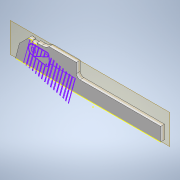
# Autodesk Inventor part: FINALcASEING
Saved by Autodesk Inventor 2022 (Build 260153000, 153)
## iProperties
Created: 2022-05-17
Part Number: FINALcASEING
Material: Generic
Document SubType Name: Sheet Metal
Designer: joshn
Density: 1 g/cm^3
Sheet Metal Rule: Default
Appearance: Default
Author: joshn
Autodesk Inventor part; units mm, degrees
ref_plane "YZ Plane" through (0, 0, 0) normal (1, 0, 0) x (0, 1, 0)
ref_plane "XZ Plane" through (0, 0, 0) normal (0, 1, 0) x (-1, 0, 0)
ref_plane "XY Plane" through (0, 0, 0) normal (0, 0, 1) x (1, 0, 0)
sketch "Sketch1" plane through (0, 0, 0) normal (0, 0, 1) x (1, 0, 0)
  line L0 (26.0925, 1.395) -> (-29.8488, 1.395)
  line L1 (26.0925, 6.611) -> (26.0925, 1.395)
  line L2 (-4.9967, 6.611) -> (26.0925, 6.611)
  arc A0 (-6.3815, 7.9958) -> (-4.9967, 6.611) centre (-4.9967, 7.9958) ccw
  line L3 (-6.3815, 11.7522) -> (-6.3815, 7.9958)
  arc A1 (2.6948, 11.4852) -> (3.6377, 11.1665) centre (3.6377, 12.7207) ccw
  line L4 (28.1816, 11.1665) -> (3.6377, 11.1665)
  arc A2 (28.1816, 11.1665) -> (28.7773, 11.4852) centre (28.1816, 11.8825) ccw
  line L5 (33.3358, 11.4852) -> (28.7773, 11.4852)
  line L6 (33.3358, 4.3481) -> (33.3358, 11.4852)
  line L7 (31.5081, -0.0048) -> (33.3358, 4.3481)
  line L8 (6.4399, -0.0048) -> (31.5081, -0.0048)
  arc A3 (6.4399, -0.0048) -> (0.2019, -8.5692) centre (6.4399, -6.5588) ccw
  arc A4 (-0.2259, -9.1565) -> (0.2019, -8.5692) centre (-0.2259, -8.7071) ccw
  line L9 (-8.1638, -9.1565) -> (-0.2259, -9.1565)
  line L10 (-9.2556, -8.793) -> (-8.1638, -9.1565)
  arc A5 (-9.2556, -8.793) -> (-11.9702, -10.6446) centre (-9.6874, -11.0757) ccw
  line L11 (-14.0648, -21.738) -> (-11.9702, -10.6446)
  arc A6 (-14.0648, -21.738) -> (-13.9231, -23.1489) centre (-11.5297, -22.1959) ccw
  line L12 (-12.9221, -25.6631) -> (-13.9231, -23.1489)
  line L13 (-29.6181, -25.6631) -> (-12.9221, -25.6631)
  line L14 (-30.9465, -25.0614) -> (-29.6181, -25.6631)
  line L15 (-31.1458, -21.5976) -> (-30.9465, -25.0614)
  arc A7 (-30.2453, -17.6448) -> (-31.1458, -21.5976) centre (-23.86, -21.1784) ccw
  arc A8 (-30.2453, -17.6448) -> (-27.8942, -12.0594) centre (-55.0684, -3.9079) ccw
  line L16 (-26.4293, -7.1761) -> (-27.8942, -12.0594)
  arc A9 (-26.4293, -7.1761) -> (-31.0096, -1.0202) centre (-31.0096, -5.8021) ccw
  line L17 (-36.2536, -1.0202) -> (-31.0096, -1.0202)
  arc A10 (-36.381, -0.6693) -> (-36.2536, -1.0202) centre (-36.2536, -0.8216) ccw
  arc A11 (-31.0437, 1.6032) -> (-36.381, -0.6693) centre (-29.9586, -8.349) ccw
  line L18 (-28.3022, 7.1894) -> (-29.8488, 1.395)
  arc A12 (-8.4832, -1.7741) -> (-7.3734, -1.1742) centre (-9.8084, 2.0038) ccw
  arc A13 (-8.4832, -1.7741) -> (-9.7826, -7.4755) centre (-7.34, -5.0334) ccw
  arc A14 (-9.7826, -7.4755) -> (-7.6044, -8.3792) centre (-7.6013, -5.2947) ccw
  line L19 (-7.6044, -8.3792) -> (-2.3274, -8.3792)
  arc A15 (-2.3274, -8.3792) -> (-1.0505, -7.1023) centre (-2.3274, -7.1023) ccw
  line L20 (-1.0505, -7.1023) -> (-1.0505, -4.8739)
  arc A16 (-1.0505, -4.8739) -> (-4.9041, -1.0202) centre (-4.9041, -4.8739) ccw
  line L21 (-4.9041, -1.0202) -> (-6.9193, -1.0202)
  arc A17 (-6.9193, -1.0202) -> (-7.3734, -1.1742) centre (-6.9193, -1.767) ccw
  arc A18 (-19.7638, 10.6339) -> (-16.9019, 11.7522) centre (-19.7638, 14.8551) ccw
  line L22 (-6.3815, 11.7522) -> (-16.9019, 11.7522)
  line L23 (-19.7638, 10.6339) -> (-21.6251, 10.6339)
  line L24 (-23.3493, 10.6339) -> (-24.8791, 10.6339)
  line L25 (-24.8791, 10.6339) -> (-28.3022, 7.1894)
  line L26 (-23.3493, 10.6339) -> (-23.7221, 10.0493)
  line L27 (-23.7221, 10.0493) -> (-21.2622, 10.0493)
  line L28 (-21.2622, 10.0493) -> (-21.6251, 10.6339)
  point P0 (0, 0)
extrude "Plate1" add sketch "Sketch1" along normal blind 1.5 contours L0 L18 L25 L24 L26 L27 L28 L23 A18 L22 L3 A0 L2 L1
sketch "Sketch2" plane through (0, 0, 1.5) normal (0, 0, 1) x (1, 0, 0)
  line L0 (-24.8791, 10.6339) -> (-23.3493, 10.6339) projected
  line L1 (-24.2815, 10.6339) -> (-26.8252, 1.395)
  line L2 (26.0925, 1.395) -> (-29.8488, 1.395) projected
  line L3 (-16.1938, 8.4071) -> (-18.7375, -0.8317)
  line L4 (-15.9942, 8.3522) -> (-18.5379, -0.8867)
  line L5 (-15.2196, 8.1389) -> (-17.7634, -1.1)
  line L6 (-14.9385, 8.0615) -> (-17.4822, -1.1774)
  line L7 (-13.9643, 7.7933) -> (-16.5081, -1.4456)
  line L8 (-13.7067, 7.7224) -> (-16.2504, -1.5165)
  line L9 (-12.8263, 7.48) -> (-15.37, -1.7589)
  line L10 (-12.5495, 7.4038) -> (-15.0932, -1.8351)
  line L11 (-11.612, 7.1457) -> (-14.1558, -2.0932)
  line L12 (-11.4028, 7.0881) -> (-13.9465, -2.1508)
  line L13 (-10.3931, 6.8101) -> (-12.9369, -2.4288)
  line L14 (-10.137, 6.7395) -> (-12.6808, -2.4993)
  line L15 (-9.1755, 6.4748) -> (-11.7192, -2.7641)
  line L16 (-8.9034, 6.3999) -> (-11.4471, -2.839)
  line L17 (-8.1272, 6.2147) -> (-10.7056, -3.1502)
  line L18 (-7.8808, 6.2147) -> (-10.4766, -3.2133)
  line L19 (-6.8145, 6.2147) -> (-9.4855, -3.4861)
  line L20 (-6.9417, 6.2147) -> (-9.6037, -3.4536)
  arc A0 (-22.976, 9.5181) -> (-23.3371, 5.5802) centre (-23.0061, 7.5354) ccw
  line L21 (-22.976, 9.5181) -> (-17.7655, 9.5181)
  arc A1 (-16.95, 8.7307) -> (-17.7655, 9.5181) centre (-17.7655, 8.7021) ccw
  line L22 (-16.95, 8.7307) -> (-16.8802, 6.7415)
  line L23 (-16.8802, 6.7415) -> (-17.3174, 5.1538)
  arc A2 (-18.0525, 4.6855) -> (-17.3174, 5.1538) centre (-17.944, 5.3263) ccw
  line L24 (-18.0525, 4.6855) -> (-23.3371, 5.5802)
  circle A3 centre (-23.0061, 7.5354) radius 0.8711
  arc A4 (-23.0061, 9.3529) -> (-22.235, 5.8895) centre (-23.0061, 7.5354) ccw
  line L25 (-23.0061, 9.3529) -> (-17.7655, 9.3529)
  arc A5 (-17.4894, 8.1128) -> (-17.7655, 9.3529) centre (-17.7655, 8.7021) ccw
  line L26 (-17.4894, 8.1128) -> (-22.235, 5.8895)
  line L27 (-6.8145, 6.2147) -> (-17.0253, 6.2147)
  line L28 (-23.3493, 10.6339) -> (-23.7221, 10.0493) projected
  line L29 (-23.7221, 10.0493) -> (-21.2622, 10.0493) projected
  line L30 (-22.2015, 5.818) -> (-17.4559, 8.0413)
  arc A6 (-17.4559, 8.0413) -> (-17.7655, 9.4318) centre (-17.7655, 8.7021) ccw
  line L31 (-17.7655, 9.4318) -> (-23.0061, 9.4318)
  arc A7 (-23.0061, 9.4318) -> (-22.2015, 5.818) centre (-23.0061, 7.5354) ccw
  line L32 (-22.9381, 6.6239) -> (-23.0741, 6.6239)
  line L33 (-23.0741, 6.6239) -> (-23.0741, 8.4468)
  line L34 (-23.0741, 8.4468) -> (-22.9381, 8.4468)
  line L35 (-22.9381, 8.4468) -> (-22.9381, 6.6239)
  line L36 (-22.9381, 6.6239) -> (-23.0741, 8.4468) construction
  line L37 (-23.0741, 6.6239) -> (-22.9381, 8.4468) construction
  line L38 (-23.2868, 10.36) -> (-23.5907, 9.2563)
  line L39 (-23.0483, 10.2944) -> (-23.858, 7.3534)
  line L40 (-24.3892, 6.3561) -> (-24.4143, 6.265)
  line L41 (-24.4413, 6.1669) -> (-25.8305, 1.1212)
  line L42 (-24.188, 6.1546) -> (-24.2111, 6.0709)
  line L43 (-24.2361, 5.9799) -> (-25.592, 1.0555)
  line L44 (-22.1805, 10.0555) -> (-23.386, 5.6773)
  line L45 (-23.409, 5.5937) -> (-24.7242, 0.8166)
  line L46 (-21.9016, 9.9786) -> (-23.0959, 5.641)
  line L47 (-23.1226, 5.5439) -> (-24.4453, 0.7398)
  line L48 (-20.9546, 9.7179) -> (-22.0026, 5.9112)
  line L49 (-22.1492, 5.379) -> (-23.4983, 0.479)
  line L50 (-20.7608, 9.6646) -> (-21.7633, 6.0233)
  line L51 (-21.95, 5.3453) -> (-23.3045, 0.4257)
  line L52 (-19.7243, 9.3792) -> (-20.4831, 6.6231)
  line L53 (-20.8846, 5.1649) -> (-22.268, 0.1403)
  line L54 (-19.5731, 9.3375) -> (-20.2963, 6.7106)
  line L55 (-20.7291, 5.1386) -> (-22.1168, 0.0987)
  line L56 (-18.6217, 9.0756) -> (-19.1213, 7.261)
  line L57 (-19.7513, 4.9731) -> (-21.1654, -0.1633)
  line L58 (-18.3758, 9.0079) -> (-18.8176, 7.4034)
  line L59 (-19.4985, 4.9303) -> (-20.9195, -0.231)
  line L60 (-17.4405, 8.7504) -> (-17.6623, 7.9446)
  line L61 (-18.5371, 4.7675) -> (-19.9842, -0.4885)
  line L62 (-17.243, 8.696) -> (-17.418, 8.0604)
  line L63 (-18.3341, 4.7331) -> (-19.7867, -0.5429)
  arc A8 (-22.9763, 9.4848) -> (-23.3316, 5.6131) centre (-23.0061, 7.5354) ccw
  line L64 (-22.9763, 9.4848) -> (-17.7655, 9.4848)
  arc A9 (-16.9833, 8.7295) -> (-17.7655, 9.4848) centre (-17.7655, 8.7021) ccw
  line L65 (-16.9833, 8.7295) -> (-16.9137, 6.7454)
  line L66 (-16.9137, 6.7454) -> (-17.3495, 5.1626)
  arc A10 (-18.0469, 4.7184) -> (-17.3495, 5.1626) centre (-17.944, 5.3263) ccw
  line L67 (-18.0469, 4.7184) -> (-23.3316, 5.6131)
  point P0 (0, 0)
  point P1 (-9.2078, 1.395)
  point P2 (-8.2687, 1.395)
  point P3 (-8.9543, 6.2147)
  point P4 (-10.2813, 1.395)
  point P5 (-9.4541, 1.395)
  point P6 (-9.2471, 6.2147)
  point P7 (-10.2815, 6.2147)
  point P8 (-11.6085, 1.395)
  point P9 (-10.5741, 1.395)
  point P10 (-10.5571, 6.2147)
  point P11 (-11.6433, 6.2147)
  point P12 (-12.9703, 1.395)
  point P13 (-11.8841, 1.395)
  point P14 (-11.8684, 6.2147)
  point P15 (-12.8769, 6.2147)
  point P16 (-14.2039, 1.395)
  point P17 (-13.1954, 1.395)
  point P18 (-13.1747, 6.2147)
  point P19 (-14.1218, 6.2147)
  point P20 (-15.4488, 1.395)
  point P21 (-14.5017, 1.395)
  point P22 (-14.399, 6.2147)
  point P23 (-15.447, 6.2147)
  point P24 (-16.774, 1.395)
  point P25 (-15.726, 1.395)
  point P26 (-15.7494, 6.2147)
  point P27 (-16.5827, 6.2147)
  point P28 (-17.9097, 1.395)
  point P29 (-17.0764, 1.395)
  point P30 (-18.1244, 1.395)
  point P31 (-16.7974, 6.2147)
  point P32 (-23.0061, 7.5354)
  point P33 (-22.9381, 8.4038)
  point P34 (-22.9381, 6.6669)
  point P35 (-23.0741, 8.4038)
  point P36 (-23.0741, 6.6669)
  point P37 (-8.1415, 1.395)
  point P38 (-19.2531, 1.395)
  point P39 (-19.4656, 1.395)
  point P40 (-20.4718, 1.395)
  point P41 (-20.7364, 1.395)
  point P42 (-21.7598, 1.395)
  point P43 (-21.9225, 1.395)
  point P44 (-23.0376, 1.395)
  point P45 (-23.2461, 1.395)
  point P46 (-24.2649, 1.395)
  point P47 (-24.565, 1.395)
  point P48 (-25.4985, 1.395)
  point P49 (-25.7551, 1.395)
  point P50 (-23.5386, 9.4455)
  point P51 (-23.3723, 10.0493)
  point P52 (-20.8103, 9.4848)
  point P53 (-20.8248, 9.4318)
  point P54 (-23.5656, 9.3474)
  point P55 (-23.5489, 9.4079)
  constraints: 124 end point, 77 parallel, 31 point on circle, 10 centre point, 7 tangent, 5 point on line, 3 horizontal, 2 coincident, 2 midpoint, 1 concentric, 1 perpendicular, 38 other
extrude "Extrusion1" cut sketch "Sketch2" against normal blind 0.1 contours L0 L28 L29 L38 A0 L41 L2 L1 | L43 A0 L45 L2 | L47 L24 L49 L2 | L51 L24 L53 L2 | L55 L24 L57 L2 | L59 L24 L61 L2 | L27 L3 L2 L63 L24 A2 L23 | L27 L5 L2 L4 | L27 L7 L2 L6 | L27 L9 L2 L8 | L27 L11 L2 L10 | L27 L13 L2 L12 | L27 L15 L2 L14 | L27 L17 L2 L16 | L27 L20 L2 L18
extrude "Extrusion4" cut sketch "Sketch2" against normal blind 0.1 contours L38 A4 L40 A7 | A7 L39 A4 L38 | A7 L31 L44 L25 A4 L39 | L40 A4 L42 A7 | L31 L46 L25 L44 | L42 A4 L44 A7 | L31 L48 L25 L46 | L44 A4 L46 A7 | L31 L50 L25 L48 | L46 A4 L26 L48 L30 A7 | L31 A6 L62 A5 L25 L50 | L26 L50 L30 L48 | A6 L30 L60 L26 A5 L62 | L26 L52 L30 L50 | L26 L54 L30 L52 | L30 L58 L26 L60 | L26 L56 L30 L54 | L30 L56 L26 L58
extrude "Extrusion5" cut sketch "Sketch2" against normal blind 0.1 contours L39 A3 | A3 L33 L44 L39 | L44 L35 A3 | A3 L46 L35 L44 | A3 L46 | L33 A3 L44
extrude "Extrusion6" cut sketch "Sketch2" against normal blind 0.1 contours L38 A7 L30 A6 L31 L50 L64 A9 L65 L66 A10 L67 A8
ref_plane "Work Plane1" through (0, 0, 0.75) normal (0, 0, 1) x (1, 0, 0)
mirror "Mirror1" about plane through (0, 0, 0.75) normal (0, 0, 1) of "Extrusion1", "Extrusion4", "Extrusion5", "Extrusion6"
equation "\"d0\" = Thickness"
equation "\"BendRadius\" = Thickness"
equation "\"BendReliefWidth\" = Thickness"
equation "\"BendReliefDepth\" = 0.5 * Thickness"
equation "\"CornerReliefSize\" = 4 * Thickness"
equation "\"MinimumRemnant\" = 2 * Thickness"
equation "\"TransitionRadius\" = BendRadius"
equation "\"JacobiRadiusSize\" = BendRadius"
equation "\"GapSize\" = Thickness"
equation "\"Thickness\" = 1.5"
body "Solid1"
